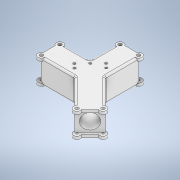
# Autodesk Inventor part: shockMount
Saved by Autodesk Inventor 2022 (Build 260153000, 153)
## iProperties
Created: 2022-02-09
Part Number: shockMount
Material: Generic
Document SubType Name: Modeling
Designer: ultra
Density: 1 g/cm^3
Appearance: Smooth - White
Author: ultra
Autodesk Inventor part; units mm, degrees
ref_plane "YZ Plane" through (0, 0, 0) normal (1, 0, 0) x (0, 1, 0)
ref_plane "XZ Plane" through (0, 0, 0) normal (0, 1, 0) x (-1, 0, 0)
ref_plane "XY Plane" through (0, 0, 0) normal (0, 0, 1) x (1, 0, 0)
sketch "Sketch1" plane through (0, 0, 0) normal (1, 0, 0) x (0, 1, 0)
  line L0 (0, 0) -> (41.5544, 0)
  line L1 (41.5544, 0) -> (41.5544, 37.0078)
  line L2 (41.5544, 37.0078) -> (0, 37.0078)
  line L3 (0, 37.0078) -> (0, 0)
  circle A0 centre (20.7772, 18.5039) radius 12.8778
  dimension "d0" = 41.5544
  dimension "d1" = 37.0078
  dimension "d2" = 25.7556
  constraints: 8 end point, 2 parallel, 1 centre point, 1 horizontal, 1 perpendicular
  measures "d0" distance of L2.end L1.end
  measures "d1" distance of L1.end L0.end
  measures "d2" diameter of A0
extrude "Extrusion1" add sketch "Sketch1" along normal blind 50.8
sketch "Sketch2" plane through (0, 0, 0) normal (0, 0, -1) x (-1, 0, 0)
  line L0 (-50.8, 0) -> (-50.8, 41.5544) projected
  line L1 (-50.8, 41.5544) -> (-87.8078, 41.5544)
  line L2 (-87.8078, 41.5544) -> (-87.8078, 0)
  line L3 (-87.8078, 0) -> (-50.8, 0)
  line L4 (-50.8, 0) -> (-50.8, 41.5544)
  circle A0 centre (-69.3039, 20.7772) radius 12.8778
  dimension "d5" = 37.0078
  dimension "d6" = 25.7556
  constraints: 8 end point, 2 parallel, 1 centre point, 1 horizontal, 1 perpendicular
  measures "d5" distance of L3.end L2.end
  measures "d6" diameter of A0
extrude "Extrusion2" add sketch "Sketch2" against normal up to surface (37.0078 mm away) contours L3 L2 L1 L0 | A0
sketch "Sketch3" plane through (0, 0, 0) normal (0, 0, -1) x (-1, 0, 0)
  line L0 (0, 41.5544) -> (-87.8078, 41.5544) projected
  line L1 (-87.8078, 41.5544) -> (-87.8078, 0) projected
  line L2 (0, 0) -> (-87.8078, 0) projected
  line L3 (0, 0) -> (-87.8078, 0) projected
  line L4 (-87.8078, 41.5544) -> (-50.8, 41.5544)
  line L5 (-50.8, 41.5544) -> (-50.8, 0)
  line L6 (-50.8, 0) -> (-87.8078, 0)
  line L7 (-87.8078, 0) -> (-87.8078, 41.5544)
  circle A0 centre (-69.3039, 20.7772) radius 12.8778
  point P0 (-50.8, 0)
  dimension "d9" = 37.0078
  dimension "d10" = 25.7556
  constraints: 8 end point, 2 parallel, 1 centre point, 1 horizontal, 1 perpendicular, 1 point on line
  measures "d9" distance of L5.end L6.end
  measures "d10" diameter of A0
extrude "Extrusion3" add sketch "Sketch3" along normal blind 50.8
sketch "Sketch4" plane through (0, 41.5544, 37.0078) normal (0, 1, 0) x (1, 0, 0)
  line L0 (0, 0) -> (87.8078, 0)
  line L1 (87.8078, 87.8078) -> (87.8078, 0)
  line L2 (50.8, 37.0078) -> (50.8, 87.8078)
  line L3 (87.8078, 0) -> (87.8078, 87.8078)
  line L4 (50.8, 37.0078) -> (87.8078, 0)
  line L5 (87.8078, 0) -> (123.159418, -36.481545)
  line L6 (87.8078, 0) -> (100.892033, 13.084233)
  line L7 (0, 0) -> (87.8078, 0)
  line L8 (87.8078, 0) -> (74.723567, -13.084233)
  line L9 (100.892033, 13.084233) -> (87.8078, 26.168466)
  line L10 (74.723567, -13.084233) -> (61.639334, 0)
  line L11 (100.892033, 13.084233) -> (136.808615, -22.832348)
  line L12 (136.808615, -22.832348) -> (123.159418, -36.481545)
  line L13 (123.159418, -36.481545) -> (110.640148, -49.000815)
  line L14 (123.159418, -36.481545) -> (140.864338, -36.481545) construction
  line L15 (110.640148, -49.000815) -> (74.723567, -13.084233)
  dimension "d13" = 50.8
  dimension "d14" = 18.5039
  dimension "d15" = 18.5039
  dimension "d16" = 135
  constraints: 22 end point, 4 point on line, 3 perpendicular, 1 equal length, 1 horizontal
  measures "d13" distance of L0.end L5.end
  measures "d14" distance of L0.end L6.end
  measures "d15" distance of L0.end L8.end
  measures "d16" angle of L13 L14
extrude "Extrusion4" add sketch "Sketch4" against normal up to surface (41.5544 mm away)
sketch "Sketch5" plane through (136.808615, 0, 59.840148) normal (0.7071068, 0, 0.7071068) x (0.7071068, 0, -0.7071068)
  line L0 (-18.5039, 41.5544) -> (-18.5039, 0) projected
  circle A0 centre (-18.5039, 20.7772) radius 12.8778
  point P0 (-54.424924, 0)
  dimension "d19" = 25.7556
  constraints: 1 centre point, 1 midpoint
  measures "d19" diameter of A0
extrude "Extrusion5" cut sketch "Sketch5" against normal blind 76.2
sketch "Sketch6" plane through (0, 41.5544, 37.0078) normal (0, 1, 0) x (1, 0, 0)
  line L0 (0, 37.0078) -> (0, 0)
  line L1 (0, 0) -> (61.639334, 0)
  line L2 (61.639334, 0) -> (110.640148, -49.000815)
  line L3 (110.640148, -49.000815) -> (136.808615, -22.832348)
  line L4 (136.808615, -22.832348) -> (87.8078, 26.168466)
  line L5 (87.8078, 87.8078) -> (87.8078, 26.168466)
  line L6 (50.8, 87.8078) -> (87.8078, 87.8078)
  line L7 (50.8, 37.0078) -> (50.8, 87.8078)
  line L8 (0, 37.0078) -> (50.8, 37.0078)
  line L9 (0, 18.5039) -> (69.3039, 18.5039)
  line L10 (69.3039, 18.5039) -> (69.3039, 87.8078)
  line L11 (56.4261, 87.8078) -> (82.1817, 87.8078)
  line L12 (69.3039, 18.5039) -> (123.724381, -35.916581)
  circle A0 centre (2.4892, 2.879001) radius 1.5875
  circle A1 centre (2.4892, 34.128799) radius 1.5875
  circle A2 centre (84.928799, 85.3186) radius 1.5875
  circle A3 centre (53.679001, 85.3186) radius 1.5875
  circle A4 centre (110.915779, -45.204923) radius 1.5875
  circle A5 centre (133.012723, -23.107979) radius 1.5875
  dimension "d22" = 3.175
  dimension "d23" = 3.175
  dimension "d24" = 2.4892
  dimension "d25" = 2.4892
  dimension "d26" = 2.879
  dimension "d27" = 2.879
  dimension "d28" = 3.175
  dimension "d29" = 3.175
  dimension "d30" = 2.4892
  dimension "d31" = 2.4892
  dimension "d32" = 2.879
  dimension "d33" = 2.879
  dimension "d34" = 3.175
  dimension "d35" = 3.175
  dimension "d36" = 2.4892
  dimension "d37" = 2.4892
  dimension "d38" = 2.879
  dimension "d39" = 2.879
  constraints: 6 centre point, 6 end point, 3 midpoint, 1 perpendicular
  measures "d22" diameter of A0
  measures "d23" diameter of A1
  measures "d24" distance from line of L0 A0.centre
  measures "d25" distance from line of L0 A1.centre
  measures "d26" distance from line of L1 A0.centre
  measures "d27" distance from line of L8 A1.centre
  measures "d28" diameter of A2
  measures "d29" diameter of A3
  measures "d30" vertical distance of L11.start A3.centre
  measures "d31" distance from line of L6 A2.centre
  measures "d32" distance from line of L5 A2.centre
  measures "d33" distance from line of L7 A3.centre
  measures "d34" diameter of A4
  measures "d35" diameter of A5
  measures "d36" distance from line of L3 A4.centre
  measures "d37" distance from line of L3 A5.centre
  measures "d38" distance from line of L4 A5.centre
  measures "d39" distance from line of L2 A4.centre
extrude "Extrusion6" cut sketch "Sketch6" against normal blind 50.8 contours A0 | A1 | A2 | A3 | A4 | A5
sketch "Sketch7" plane through (0, 41.5544, 37.0078) normal (0, 1, 0) x (1, 0, 0)
  circle A0 centre (2.4892, 2.879001) radius 1.5875
  circle A1 centre (110.915779, -45.204923) radius 1.5875
  circle A2 centre (53.679001, 85.3186) radius 1.5875
  circle A3 centre (2.4892, 34.128799) radius 1.5875
  circle A4 centre (84.928799, 85.3186) radius 1.5875
  line L0 (0, 37.0078) -> (0, 0)
  line L1 (0, 0) -> (61.639334, 0)
  line L2 (61.639334, 0) -> (110.640148, -49.000815)
  line L3 (110.640148, -49.000815) -> (136.808615, -22.832348)
  line L4 (136.808615, -22.832348) -> (87.8078, 26.168466)
  line L5 (87.8078, 87.8078) -> (87.8078, 26.168466)
  line L6 (50.8, 87.8078) -> (87.8078, 87.8078)
  line L7 (50.8, 37.0078) -> (50.8, 87.8078)
  line L8 (0, 37.0078) -> (50.8, 37.0078)
  circle A5 centre (133.012723, -23.107979) radius 1.5875
  circle A6 centre (133.012723, -23.107979) radius 6
  circle A7 centre (110.915779, -45.204923) radius 6
  circle A8 centre (2.4892, 2.879001) radius 6
  circle A9 centre (2.4892, 34.128799) radius 6
  circle A10 centre (53.679001, 85.3186) radius 6
  circle A11 centre (84.928799, 85.3186) radius 6
  point P0 (0, 8.338294)
  point P1 (7.753357, 0)
  point P2 (7.753357, 37.0078)
  point P3 (0, 28.669506)
  point P4 (59.138294, 87.8078)
  point P5 (50.8, 80.054443)
  point P6 (79.469506, 87.8078)
  point P7 (87.8078, 80.054443)
  point P8 (130.91255, -28.728413)
  point P9 (131.326163, -17.349897)
  point P10 (105.157697, -43.518363)
  point P11 (116.536213, -43.10475)
  dimension "d42" = 12
  dimension "d43" = 12
  dimension "d44" = 12
  dimension "d45" = 12
  dimension "d46" = 12
  dimension "d47" = 12
  constraints: 6 centre point, 6 coincident
  measures "d42" diameter of A6
  measures "d43" diameter of A7
  measures "d44" diameter of A8
  measures "d45" diameter of A9
  measures "d46" diameter of A10
  measures "d47" diameter of A11
extrude "Extrusion7" add sketch "Sketch7" against normal blind 4.7752 contours L0 A9 L8 | L0 L1 A8 | A10 L6 L7 | L2 L3 A7 | A11 L5 L6 | L3 L4 A6 picked at (-0.40329, 31.69401) picked at (-0.40329, 5.31379) picked at (56.11379, 88.21109) picked at (106.906155, -45.827693) picked at (82.506669, 88.227088) picked at (133.345386, -26.876011)
sketch "Sketch8" plane through (0, 0, 0) normal (0, -1, 0) x (1, 0, 0)
  circle A0 centre (2.4892, 34.128799) radius 1.5875
  circle A1 centre (53.679001, -48.3108) radius 1.5875
  circle A2 centre (2.4892, 2.879001) radius 1.5875
  circle A3 centre (84.928799, -48.3108) radius 1.5875
  line L0 (0, 37.0078) -> (0, 0)
  line L1 (0, 0) -> (50.8, 0)
  line L2 (50.8, 0) -> (50.8, -50.8)
  line L3 (87.8078, -50.8) -> (50.8, -50.8)
  line L4 (87.8078, 10.839334) -> (87.8078, -50.8)
  line L5 (136.808615, 59.840148) -> (87.8078, 10.839334)
  line L6 (110.640148, 86.008615) -> (136.808615, 59.840148)
  line L7 (61.639334, 37.0078) -> (110.640148, 86.008615)
  line L8 (0, 37.0078) -> (61.639334, 37.0078)
  circle A4 centre (110.915779, 82.212723) radius 1.5875
  circle A5 centre (110.915779, 82.212723) radius 6
  circle A6 centre (133.012723, 60.115779) radius 1.5875
  circle A7 centre (133.012723, 60.115779) radius 6
  circle A8 centre (84.928799, -48.3108) radius 6
  circle A9 centre (53.679001, -48.3108) radius 6
  circle A10 centre (2.4892, 2.879001) radius 6
  circle A11 centre (2.4892, 34.128799) radius 6
  point P0 (0, 8.338294)
  point P1 (7.753357, 0)
  point P2 (7.753357, 37.0078)
  point P3 (0, 28.669506)
  point P4 (116.536213, 80.11255)
  point P5 (105.157697, 80.526163)
  point P6 (131.326163, 54.357697)
  point P7 (130.91255, 65.736213)
  point P8 (87.8078, -43.046643)
  point P9 (79.469506, -50.8)
  point P10 (50.8, -43.046643)
  point P11 (59.138294, -50.8)
  dimension "d50" = 12
  constraints: 6 centre point, 6 coincident
  measures "d50" diameter of A5
extrude "Extrusion8" add sketch "Sketch8" against normal blind 4.7752 contours L0 A11 L8 | L0 L1 A10 | A5 L6 L7 | L2 L3 A9 | A7 L5 L6 | L3 L4 A8 picked at (-0.40329, 31.69401) picked at (-0.40329, 5.31379) picked at (106.906155, 82.835493) picked at (56.11379, -51.20329) picked at (133.345386, 63.883811) picked at (82.506669, -51.219288)
sketch "Sketch9" plane through (0, 41.5544, 28.669506) normal (0, 1, 0) x (1, 0, 0)
  circle A0 centre (2.4892, -5.459293) radius 1.5875
  circle A1 centre (110.915779, -53.543218) radius 1.5875
  circle A2 centre (53.679001, 76.980306) radius 1.5875
  circle A3 centre (2.4892, 25.790504) radius 1.5875
  circle A4 centre (133.012723, -31.446274) radius 1.5875
  circle A5 centre (84.928799, 76.980306) radius 1.5875
  arc A6 (0, 0) -> (7.753357, -8.338294) centre (2.4892, -5.459293) ccw
  arc A7 (105.157697, -51.856657) -> (116.536213, -51.443044) centre (110.915779, -53.543218) ccw
  arc A8 (87.8078, 71.716148) -> (79.469506, 79.469506) centre (84.928799, 76.980306) ccw
  arc A9 (7.753357, 28.669506) -> (0, 20.331211) centre (2.4892, 25.790504) ccw
  circle A10 centre (110.915779, -53.543218) radius 2.925
  circle A11 centre (133.012723, -31.446274) radius 1.5875
  circle A12 centre (133.012723, -31.446274) radius 2.925
  circle A13 centre (84.928799, 76.980306) radius 2.925
  circle A14 centre (53.679001, 76.980306) radius 1.5875
  circle A15 centre (53.679001, 76.980306) radius 2.925
  circle A16 centre (2.4892, 25.790504) radius 2.925
  circle A17 centre (2.4892, -5.459293) radius 2.925
  point P0 (0, 28.669506)
  dimension "d53" = 5.85
  dimension "d54" = 5.85
  dimension "d55" = 5.85
  dimension "d56" = 5.85
  dimension "d57" = 5.85
  dimension "d58" = 5.85
  constraints: 6 centre point, 6 coincident
  measures "d53" diameter of A10
  measures "d54" diameter of A12
  measures "d55" diameter of A13
  measures "d56" diameter of A15
  measures "d57" diameter of A16
  measures "d58" diameter of A17
sketch "Sketch10" plane through (0, 0, -50.8) normal (0, 0, -1) x (-1, 0, 0)
  line L0 (-59.138294, 4.7752) -> (-50.8, 4.7752)
  line L1 (-50.8, 4.7752) -> (-50.8, 36.7792)
  line L2 (-50.8, 36.7792) -> (-59.138294, 36.7792)
  line L3 (-79.469506, 36.7792) -> (-87.8078, 36.7792)
  line L4 (-87.8078, 36.7792) -> (-87.8078, 4.7752)
  line L5 (-87.8078, 4.7752) -> (-79.469506, 4.7752)
  circle A0 centre (-69.3039, 20.7772) radius 12.8778
  line L6 (-87.8078, 4.7752) -> (-50.8, 4.7752)
  line L7 (-50.8, 4.7752) -> (-50.8, 36.7792)
  line L8 (-50.8, 36.7792) -> (-87.8078, 36.7792)
  line L9 (-87.8078, 36.7792) -> (-87.8078, 4.7752)
  line L10 (-87.8078, 4.7752) -> (-50.8, 36.7792) construction
  line L11 (-50.8, 4.7752) -> (-87.8078, 36.7792) construction
  point P0 (0, 0)
  constraints: 12 end point, 2 midpoint, 2 parallel, 1 horizontal, 1 perpendicular
extrude "Extrusion9" cut sketch "Sketch10" against normal blind 5.0038
sketch "Sketch11" plane through (0, 0, 0) normal (-1, 0, 0) x (0, 0, 1)
  line L0 (28.669506, 4.7752) -> (37.0078, 4.7752)
  line L1 (37.0078, 36.7792) -> (37.0078, 4.7752)
  line L2 (37.0078, 36.7792) -> (28.669506, 36.7792)
  line L3 (8.338294, 36.7792) -> (0, 36.7792)
  line L4 (0, 4.7752) -> (0, 36.7792)
  line L5 (0, 4.7752) -> (8.338294, 4.7752)
  circle A0 centre (18.5039, 20.7772) radius 12.8778
  line L6 (0, 4.7752) -> (37.0078, 4.7752)
  line L7 (37.0078, 4.7752) -> (37.0078, 36.7792)
  line L8 (37.0078, 36.7792) -> (0, 36.7792)
  line L9 (0, 36.7792) -> (0, 4.7752)
  line L10 (0, 4.7752) -> (37.0078, 36.7792) construction
  line L11 (37.0078, 4.7752) -> (0, 36.7792) construction
  point P0 (0, 0)
  constraints: 12 end point, 2 midpoint, 2 parallel, 1 horizontal, 1 perpendicular
extrude "Extrusion10" cut sketch "Sketch11" against normal blind 5.0038
sketch "Sketch12" plane through (130.91255, 36.7792, 65.736213) normal (0.7071068, 0, 0.7071068) x (0.7071068, 0, -0.7071068)
  line L0 (0, -32.004) -> (8.338294, -32.004)
  line L1 (8.338294, 0) -> (8.338294, -32.004)
  line L2 (8.338294, 0) -> (0, 0)
  line L3 (-20.331211, 0) -> (-28.669506, 0)
  line L4 (-28.669506, 0) -> (-28.669506, -32.004)
  line L5 (-28.669506, -32.004) -> (-20.331211, -32.004)
  circle A0 centre (-10.165606, -16.002) radius 12.8778
  line L6 (-28.669506, -32.004) -> (8.338294, -32.004)
  line L7 (8.338294, -32.004) -> (8.338294, 0)
  line L8 (8.338294, 0) -> (-28.669506, 0)
  line L9 (-28.669506, 0) -> (-28.669506, -32.004)
  line L10 (-28.669506, -32.004) -> (8.338294, 0) construction
  line L11 (8.338294, -32.004) -> (-28.669506, 0) construction
  point P0 (-46.08663, -36.7792)
  point P1 (-20.331211, 0)
  point P2 (-20.331211, -32.004)
  constraints: 12 end point, 2 midpoint, 2 parallel, 1 horizontal, 1 perpendicular
extrude "Extrusion11" cut sketch "Sketch12" against normal blind 5.0038
extrude "Extrusion12" cut sketch "Sketch9" against normal blind 5.08
fillet "Fillet1" radius 3.175 15 edges at (50.8, 20.7772, 0) (29.2767, 41.5544, 0) (50.8, 41.5544, -21.5233) (50.8, 0, -21.5233) (29.2767, 0, 0) (34.6963, 41.5544, 37.0078) (83.3985, 41.5544, 58.767) (83.3985, 0, 58.767) (109.567, 41.5544, 32.5985) (109.567, 0, 32.5985) (87.8078, 41.5544, -16.1037) (87.8078, 0, -16.1037) (34.6963, 0, 37.0078) (61.6393, 20.7772, 37.0078) (87.8078, 20.7772, 10.8393)
sketch "Sketch13" plane through (0, 41.5544, 28.669506) normal (0, 1, 0) x (1, 0, 0)
  line L0 (59.138294, 79.469506) -> (79.469506, 79.469506)
  line L1 (0, 20.331211) -> (0, 0)
  line L2 (116.536213, -51.443044) -> (130.91255, -37.066707)
  line L3 (78.948824, 18.732641) -> (60.736865, 0.520681)
  line L4 (79.469506, 79.469506) -> (59.138294, 79.469506)
  line L5 (69.3039, 79.469506) -> (69.3039, 9.087716)
  line L6 (69.3039, 9.087716) -> (123.185437, -44.79382)
  line L7 (130.91255, -37.066707) -> (116.536213, -51.443044)
  line L8 (0, 10.165606) -> (69.3039, 10.165606)
  circle A0 centre (15.875, 10.165606) radius 6.35
  circle A1 centre (69.3039, 63.594506) radius 6.35
  circle A2 centre (111.960117, -33.5685) radius 6.35
  circle A3 centre (41.275, 10.165606) radius 6.35
  circle A4 centre (69.3039, 38.194506) radius 6.35
  circle A5 centre (93.999604, -15.607988) radius 6.35
  circle A6 centre (76.039092, 2.352524) radius 6.35
  point P0 (0, 28.669506)
  dimension "d68" = 12.7
  dimension "d69" = 15.875
  dimension "d72" = 12.7
  dimension "d73" = 15.875
  dimension "d77" = 12.7
  dimension "d78" = 15.875
  dimension "d83" = 25.4
  dimension "d90" = 25.4
  dimension "d97" = 25.4
  constraints: 7 centre point, 6 end point, 6 point on line, 2 midpoint, 2 vertical, 1 horizontal, 1 perpendicular, 9 other
  measures "d68" diameter of A0
  measures "d69" distance from line of L1 A0.centre
  measures "d72" diameter of A1
  measures "d73" distance from line of L0 A1.centre
  measures "d77" diameter of A2
  measures "d78" distance from line of L2 A2.centre
  measures "d83" distance of A0.centre A3.centre
  measures "d90" distance of A1.centre A4.centre
  measures "d97" distance of A2.centre A5.centre
extrude "Extrusion13" [suppressed]
sketch "Sketch15" plane through (0, 0, 8.338294) normal (0, -1, 0) x (1, 0, 0)
  line L0 (0, 0) -> (0, 20.331211)
  line L1 (116.754985, -37.31401) -> (68.393487, 11.047489)
  line L2 (68.393487, 11.047489) -> (118.02233, 60.676332)
  line L3 (68.393487, 11.047489) -> (18.764644, 60.676332) construction
  line L4 (73.512233, 12.753737) -> (70.099736, 16.166235)
  line L5 (70.099736, 16.166235) -> (63.274741, 9.34124)
  line L6 (63.274741, 9.34124) -> (66.687238, 5.928743)
  line L7 (66.687238, 5.928743) -> (73.512233, 12.753737)
  line L8 (73.512233, 12.753737) -> (63.274741, 9.34124) construction
  line L9 (70.099736, 16.166235) -> (66.687238, 5.928743) construction
  line L10 (78.002361, 12.753737) -> (70.099736, 20.656363)
  line L11 (70.099736, 20.656363) -> (58.784613, 9.34124)
  line L12 (58.784613, 9.34124) -> (66.687238, 1.438615)
  line L13 (66.687238, 1.438615) -> (78.002361, 12.753737)
  line L14 (78.002361, 12.753737) -> (58.784613, 9.34124) construction
  line L15 (70.099736, 20.656363) -> (66.687238, 1.438615) construction
  point P0 (0, -8.338294)
  dimension "d104" = 90
  dimension "d105" = 4.826
  dimension "d106" = 9.652
  dimension "d107" = 11.176
  dimension "d108" = 16.002
  constraints: 30 end point, 4 midpoint, 4 parallel, 3 perpendicular
  measures "d104" angle of L2 L3
  measures "d105" distance of L6.end L5.end
  measures "d106" distance of L5.end L4.end
  measures "d107" distance of L12.end L11.end
  measures "d108" distance of L11.end L10.end
extrude "Extrusion14" add sketch "Sketch15" along normal blind 12.7 contours L13 L12 L11 L10 L2 L4 L5 L6 L7 L1 | L1 L7 L4 L2 L10 L13
sketch "Sketch16" plane through (58.784613, 0, 17.679534) normal (-0.7071068, 0, 0.7071068) x (0.7071068, 0, 0.7071068)
  line L0 (0, 0) -> (0, -12.7) projected
  line L1 (16.002, -12.7) -> (0, -12.7) projected
  circle A0 centre (8.001, -7.112) radius 3.175
  point P0 (-54.068317, 0)
  dimension "d111" = 6.35
  dimension "d112" = 8.001
  dimension "d113" = 5.588
  constraints: 1 centre point
  measures "d111" diameter of A0
  measures "d112" distance from line of L0 A0.centre
  measures "d113" distance from line of A0.centre L1
extrude "Extrusion15" cut sketch "Sketch16" against normal blind 279.4
sketch "Sketch18" plane through (0, 41.5544, 28.669506) normal (0, 1, 0) x (1, 0, 0)
  circle A0 centre (55.931223, 23.87791) radius 2.032
  circle A1 centre (49.619112, 3.536194) radius 2.032
  circle A2 centre (69.401607, 37.348294) radius 2.032
  circle A3 centre (42.744848, 10.129382) radius 2.032
  circle A4 centre (76.275871, 30.755107) radius 2.032
  point P0 (0, 28.669506)
extrude "Extrusion18" cut sketch "Sketch18" against normal blind 279.4
fillet "Fillet2" radius 6.35 4 edges at (62.7359, 0, 13.7282) (72.3448, 0, 15.4345) (74.051, 0, 25.0433) (64.4422, 0, 23.3371)
fillet "Fillet3" radius 3.175 8 edges at (66.6872, -1.8599, 7.1467) (66.6872, -9.525, 9.7769) (80.6326, -1.8599, 21.092) (78.0024, -9.525, 21.092) (70.0997, -1.8599, 31.6249) (70.0997, -9.525, 28.9947) (56.1544, -1.8599, 17.6795) (58.7846, -9.525, 17.6795)
equation "\"d7\" = d6"
body "Solid1"
